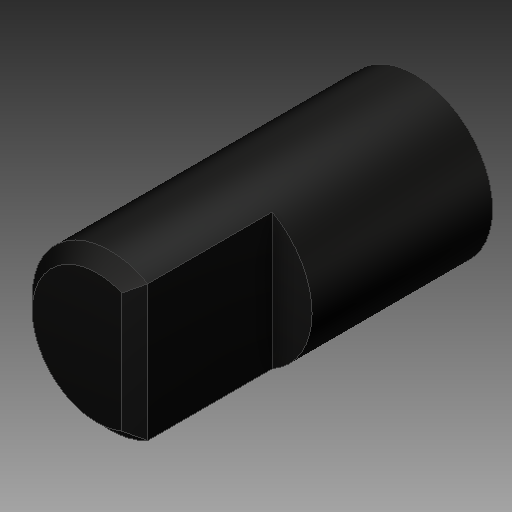
# Autodesk Inventor part: PEC12R-4017F-N0024 Shaft
Saved by Autodesk Inventor 2018 (Build 220112000, 112)
## iProperties
Created: 2018-01-11
Part Number: PEC12R-4017F-N0024 Shaft
Material: Generic
Document SubType Name: Modeling
Designer: Moochster
Density: 1 g/cm^3
Appearance: Glossy - Black
Mass: 0.314445 g
Surface Area: 2.76297 cm^2
Volume: 0.314445 cm^3
Author: Moochster
Autodesk Inventor part; units mm, degrees
ref_plane "YZ Plane" through (0, 0, 0) normal (1, 0, 0) x (0, 1, 0)
ref_plane "XZ Plane" through (0, 0, 0) normal (0, 1, 0) x (-1, 0, 0)
ref_plane "XY Plane" through (0, 0, 0) normal (0, 0, 1) x (1, 0, 0)
sketch "Sketch1" plane through (0, 0, 0) normal (0, 0, 1) x (1, 0, 0)
  circle A0 centre (0, 0) radius 3
  dimension "d0" = 6
  constraints: 1 centre point, 1 coincident
  measures "d0" diameter of A0
extrude "Extrusion1" add sketch "Sketch1" along normal blind 12.27
sketch "Sketch2" plane through (0, 0, 12.27) normal (0, 0, 1) x (1, 0, 0)
  line L0 (1.46, 2.6208) -> (1.46, -2.6208)
  circle A0 centre (0, 0) radius 3 projected
  point P0 (-3, 0)
  dimension "d3" = 4.46
  constraints: 3 point on circle, 2 end point, 1 horizontal alignment, 1 vertical
extrude "Extrusion2" cut sketch "Sketch2" against normal blind 5.3 contours A0 L0 picked at (2.441, 0.367)
chamfer "Chamfer1" distance 0.5 angle 45 2 edges at (-3, 0, 12.27) (1.46, 0, 12.27)
body "Solid1"
